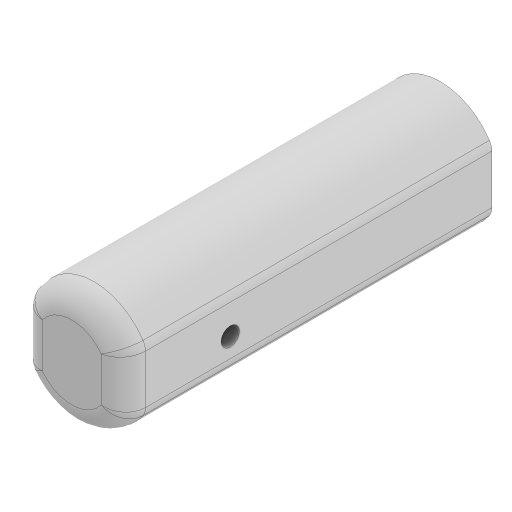
# Autodesk Inventor part: leg
Saved by Autodesk Inventor 2024 (Build 280153000, 153)
## iProperties
Created: 2023-11-07
Part Number: leg
Material: 一般
Document SubType Name: Modeling
Designer: bonju
Density: 1 g/cm^3
Appearance: 既定
Author: bonju
Autodesk Inventor part; units mm, degrees
ref_plane "YZ Plane" through (0, 0, 0) normal (1, 0, 0) x (0, 1, 0)
ref_plane "XZ Plane" through (0, 0, 0) normal (0, 1, 0) x (-1, 0, 0)
ref_plane "XY Plane" through (0, 0, 0) normal (0, 0, 1) x (1, 0, 0)
sketch "スケッチ1" plane through (0, 0, 0) normal (0, 0, 1) x (1, 0, 0)
  line L0 (0, -11.2) -> (0, 11.2) projected
  arc A0 (-7, -3.873) -> (7, -3.873) centre (0, 0) ccw
  arc A1 (7, 3.873) -> (-7, 3.873) centre (0, 0) ccw
  line L1 (-7, -3.873) -> (-7, 3.873)
  line L2 (7, -3.873) -> (7, 3.873)
  line L3 (4, 4) -> (-4, 4)
  line L4 (-4, 4) -> (-4, -4)
  line L5 (-4, -4) -> (4, -4)
  line L6 (4, -4) -> (4, 4)
  line L7 (-9.8, 0) -> (9.8, 0) projected
  dimension "d22" = 8
  dimension "d23" = 8
  dimension "d25" = 8
  dimension "d26" = 8
  dimension "d27" = 3
  constraints: 12 end point, 4 point on circle, 3 parallel, 2 centre point, 2 symmetric about line, 1 coincident, 1 horizontal, 1 perpendicular, 1 vertical, 2 other
  measures "d22" distance of L5.end L3.start
  measures "d23" distance of L3.start L3.end
  measures "d25" radius of A1
  measures "d26" radius of A0
  measures "d27" distance between parallel lines of L6 L2
extrude "押し出し1" add sketch "スケッチ1" along normal blind 50
sketch "スケッチ2" plane through (0, 0, 0) normal (0, 0, -1) x (-1, 0, 0)
  line L0 (4.05, 4.05) -> (-4.05, 4.05)
  line L1 (-4.05, 4.05) -> (-4.05, -4.05)
  line L2 (-4.05, -4.05) -> (4.05, -4.05)
  line L3 (4.05, -4.05) -> (4.05, 4.05)
  line L4 (4.05, 4.05) -> (-4.05, -4.05) construction
  line L5 (-4.05, 4.05) -> (4.05, -4.05) construction
  point P0 (0, 0)
  dimension "d28" = 8.1
  dimension "d29" = 8.1
  constraints: 12 end point, 2 midpoint, 2 parallel, 1 horizontal, 1 perpendicular
  measures "d28" distance of L2.end L1.end
  measures "d29" distance of L1.end L0.end
extrude "押し出し2" cut sketch "スケッチ2" against normal blind 5.1
sketch "スケッチ4" plane through (-7, -3.873, 0) normal (-1, 0, 0) x (0, 0, 1)
  circle A0 centre (35.5, 3.178) radius 1.25
  line L0 (50, 7.746) -> (50, 0) projected
  point P0 (0, 3.873)
  dimension "d16" = 2.5
  dimension "d17" = 14.5
  constraints: 1 centre point
  measures "d16" diameter of A0
  measures "d17" distance from line of L0 A0.centre
extrude "押し出し4" cut sketch "スケッチ4" along normal through all both and the other way through all
fillet "フィレット1" radius 3 4 edges at (0, -8, 50) (0, 8, 50) (-7, 0, 50) (7, 0, 50)
fillet "フィレット2" radius 2 8 edges at (6.0806, -3.6278, 49.1613) (7, -3.873, 23.5) (6.0806, 3.6278, 49.1613) (7, 3.873, 23.5) (-6.0806, -3.6278, 49.1613) (-7, -3.873, 23.5) (-6.0806, 3.6278, 49.1613) (-7, 3.873, 23.5)
